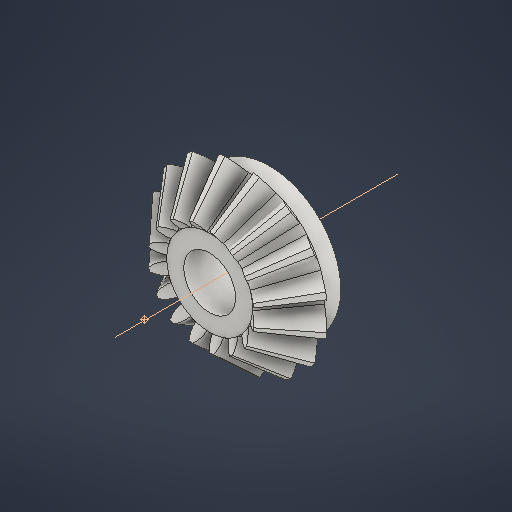
# Autodesk Inventor part: SAFRS-P-0048
Saved by Autodesk Inventor 2026.2 (Build 302298000, 298)
## iProperties
CustomPartVersion: 1
Created: 2025-11-23
Part Number: SAFRS-P-0048
Material: Steel, Mild
Document SubType Name: Modeling
Designer: jaewook
Categories: <?xml version="1.0" encoding="UTF-16"?> <MemberInstance><Categories><FamilyTemplate><FamilyTemplateParameter ValueType="xs:double" Id="1" ObjectReferenceKey="da_z" ObjectType="kUserParameterObject"/><FamilyTemplateParameter ValueType="xs:double" Id="2" ObjectReferenceKey="da_b" ObjectType="kUserParameterObject"/><FamilyTemplateParameter ValueType="xs:double" Id="3" ObjectReferenceKey="da_beta" ObjectType="kUserParameterObject"/><FamilyTemplateParameter ValueType="xs:double" Id="4" ObjectReferenceKey="da_dae" ObjectType="kUserParameterObject"/><FamilyTemplateParameter ValueType="xs:double" Id="5" ObjectReferenceKey="da_ve" ObjectType="kUserParameterObject"/><FamilyTemplateParameter ValueType="xs:double" Id="6" ObjectReferenceKey="da_omega" ObjectType="kUserParameterObject"/><FamilyTemplateParameter ValueType="xs:string" Id="7" ObjectReferenceKey="EAIAABAAAAAAHwAAAAAAAIAAAAAAAAAA" ObjectType="83914240" SubObjectId="SurfaceGeometry"/></FamilyTemplate><ParamToTemplateMap><ParamToTemplate CategoryParameter="//CategoryParameter[@InternalName='046C89C9-8512-4d59-83FE-43B91F4F132A']" TemplateParameter="1"/><ParamToTemplate CategoryParameter="//CategoryParameter[@InternalName='2552DF32-E462-4b46-AEBF-C6C7768E72AC']" TemplateParameter="2"/><ParamToTemplate CategoryParameter="//CategoryParameter[@InternalName='C9EE641D-15FC-4fae-A226-E94C4372FDD7']" TemplateParameter="3"/><ParamToTemplate><ParamToTemplate CategoryParameter="//CategoryParameter[@InternalName='00B6519A-459B-49c7-AD84-2E56D39A5744']" ConstantValue="-0.000000"/></ParamToTemplate><ParamToTemplate><ParamToTemplate CategoryParameter="//CategoryParameter[@InternalName='04B31F0E-C7A6-4894-AA32-9629BEFACF47']" ConstantValue="1.000000"/></ParamToTemplate><ParamToTemplate><ParamToTemplate CategoryParameter="//CategoryParameter[@InternalName='43CBEC2E-7847-49e7-A936-2F7889FCB2D9']" ConstantValue="0.200000"/></ParamToTemplate><ParamToTemplate><ParamToTemplate CategoryParameter="//CategoryParameter[@InternalName='B1EFC894-105D-4ebd-86BF-FA20ED196853']" ConstantValue="0.300000"/></ParamToTemplate><ParamToTemplate><ParamToTemplate CategoryParameter="//CategoryParameter[@InternalName='51175063-3D10-4879-93E8-6246FE8B403D']" ConstantValue="2060000000.000000"/></ParamToTemplate><ParamToTemplate><ParamToTemplate CategoryParameter="//CategoryParameter[@InternalName='A3A52E27-4454-46a9-B0BD-C932399B70AF']" ConstantValue="0.300000"/></ParamToTemplate><ParamToTemplate CategoryParameter="//CategoryParameter[@InternalName='2A200944-5A8C-41ca-B96E-8520D2E510F1']" TemplateParameter="4"/><ParamToTemplate><ParamToTemplate CategoryParameter="//CategoryParameter[@InternalName='1A637F62-92C8-44bc-B81F-10802510B579']" ConstantValue="1.317559"/></ParamToTemplate><ParamToTemplate CategoryParameter="//CategoryParameter[@InternalName='B52DD4BE-6863-48fb-BF58-89EF6F9EC65C']" TemplateParameter="5"/><ParamToTemplate><ParamToTemplate CategoryParameter="//CategoryParameter[@InternalName='3956BFF2-84D2-457d-93C2-9B0613DEBA67']" ConstantValue="0.703377"/></ParamToTemplate><ParamToTemplate CategoryParameter="//CategoryParameter[@InternalName='739CFA02-461B-4bf8-8049-181FCAD8B28F']" TemplateParameter="6"/><ParamToTemplate><ParamToTemplate CategoryParameter="//CategoryParameter[@InternalName='A27E999F-E2CE-4481-8A2A-EBF499C4C3C5']" ConstantValue="-0.000000"/></ParamToTemplate><ParamToTemplate><ParamToTemplate CategoryParameter="//CategoryParameter[@InternalName='9E1B4470-B2D3-4ff1-B813-535BB4CDF51A']" ConstantValue="3520000.000000"/></ParamToTemplate><ParamToTemplate><ParamToTemplate CategoryParameter="//CategoryParameter[@InternalName='F8452263-BFF6-458c-9FB1-07C4B99E95CD']" ConstantValue="11400000.000000"/></ParamToTemplate><ParamToTemplate><ParamToTemplate CategoryParameter="//CategoryParameter[@InternalName='3E3BB259-FD49-497f-8171-6EBC954A3479']" ConstantValue="2.000000"/></ParamToTemplate><ParamToTemplate CategoryParameter="//CategoryParameter[@InternalName='27C3BAF2-7550-4e4b-AE2C-0DB134B7D9B7']" TemplateParameter="7"/></ParamToTemplateMap><Category DisplayName="Gear" InternalName="DC85795E-93AB-48d5-8EEE-5A27447B64BD" Mnemonic="Gear"><CategoryParameter DisplayName="z" InternalName="046C89C9-8512-4d59-83FE-43B91F4F132A" Mnemonic="z"/><CategoryParameter DisplayName="b" InternalName="2552DF32-E462-4b46-AEBF-C6C7768E72AC" Mnemonic="b"/><CategoryParameter DisplayName="||b|" InternalName="C9EE641D-15FC-4fae-A226-E94C4372FDD7" Mnemonic="beta"/><CategoryParameter DisplayName="x" InternalName="00B6519A-459B-49c7-AD84-2E56D39A5744" Mnemonic="x"/><CategoryParameter DisplayName="a*" InternalName="04B31F0E-C7A6-4894-AA32-9629BEFACF47" Mnemonic="a"/><CategoryParameter DisplayName="c*" InternalName="43CBEC2E-7847-49e7-A936-2F7889FCB2D9" Mnemonic="c"/><CategoryParameter DisplayName="r|.f|*" InternalName="B1EFC894-105D-4ebd-86BF-FA20ED196853" Mnemonic="rf"/><CategoryParameter DisplayName="E" InternalName="51175063-3D10-4879-93E8-6246FE8B403D" Mnemonic="E"/><CategoryParameter DisplayName="||m|" InternalName="A3A52E27-4454-46a9-B0BD-C932399B70AF" Mnemonic="mi"/><Category DisplayName="BevelGear" InternalName="0C98F69A-0C2B-4791-B2FE-7691BB227E77" Mnemonic="BevelGear"><CategoryParameter DisplayName="d|.ae|" InternalName="2A200944-5A8C-41ca-B96E-8520D2E510F1" Mnemonic="dae"/><CategoryParameter DisplayName="d|.ai|" InternalName="1A637F62-92C8-44bc-B81F-10802510B579" Mnemonic="dai"/><CategoryParameter DisplayName="A|.e|" InternalName="B52DD4BE-6863-48fb-BF58-89EF6F9EC65C" Mnemonic="ve"/><CategoryParameter DisplayName="A|.i|" InternalName="3956BFF2-84D2-457d-93C2-9B0613DEBA67" Mnemonic="vi"/><CategoryParameter DisplayName="||S|" InternalName="739CFA02-461B-4bf8-8049-181FCAD8B28F" Mnemonic="omega"/><CategoryParameter DisplayName="x|.t|" InternalName="A27E999F-E2CE-4481-8A2A-EBF499C4C3C5" Mnemonic="xt"/><CategoryParameter DisplayName="||s||.Flim|" InternalName="9E1B4470-B2D3-4ff1-B813-535BB4CDF51A" Mnemonic="sFlim"/><CategoryParameter DisplayName="||s||.Hlim|" InternalName="F8452263-BFF6-458c-9FB1-07C4B99E95CD" Mnemonic="sHlim"/><CategoryParameter DisplayName="유형" InternalName="3E3BB259-FD49-497f-8171-6EBC954A3479" Mnemonic="type"/><CategoryParameter DisplayName="PitchDiameter" InternalName="27C3BAF2-7550-4e4b-AE2C-0DB134B7D9B7" Mnemonic="IDS_PITCHDIAM"/></Category></Category></Categories></MemberInstance>
Mass: 60.9118 g
Surface Area: 34.3074 cm^2
Volume: 7.7496 cm^3
Density: 7.86 g/cm^3
Appearance: Steel
Author: jaewook
Title: Bevel Gear 22T
Autodesk Inventor part; units mm, degrees
ref_plane "메쉬 평면2" through (0, 0, 0) normal (0.9807853, 0.1950903, 0) x (0, 0, 1)
sketch "톱니 본체 스케치" plane through (0, 0, 0) normal (1, 0, 0) x (0, 1, 0)
  line L0 (0, 0) -> (8.828697, -13.437043) construction
  line L1 (8.828697, -13.437043) -> (10.976086, -11.719131)
  line L2 (10.976086, -11.719131) -> (0, 0) construction
  line L3 (10, -12.5) -> (0, 0) construction
  line L4 (5.298941, -8.064848) -> (6.587794, -7.033766)
  line L5 (8.828697, -13.437043) -> (5.298941, -8.064848)
  line L6 (10.976086, -11.719131) -> (6.587794, -7.033766)
  line L7 (0, -39.386751) -> (0, 6.564458)
  line L8 (0, -12.5) -> (10.976086, -12.5) construction
  dimension "d0" = 20
  dimension "d1" = 17.65739
  dimension "d2" = 21.95217
  dimension "d3" = 6.4
  dimension "d4" = 11.71913
  constraints: 16 end point, 4 point on line, 3 perpendicular, 2 collinear, 1 horizontal alignment, 1 vertical alignment
  measures "d0" diameter of L3.start L7
  measures "d1" diameter of L0.end L7
  measures "d2" diameter of L1.end L7
  measures "d3" distance between parallel lines of L1 L4
  measures "d4" vertical distance of L1.end L0.start
revolve "톱니 본체" add sketch "톱니 본체 스케치" angle 360 about axis through (0, 0, 0) along (0, 0, 1)
ref_plane "톱니 평면" through (0, 10, -12.5) normal (0, -0.624695, 0.7808688) x (1, 0, 0)
sketch "시작 스케치" plane through (0, 10, -12.5) normal (0, -0.624695, 0.7808688) x (1, 0, 0)
  line L0 (0, -23.505131) -> (0, 10.644758)
  arc A0 (-0.541692, -1.83) -> (-2.580512, 1.849553) centre (-5.33599, -2.081868) ccw
  arc A1 (2.580512, 1.849553) -> (0.541692, -1.83) centre (5.33599, -2.081868) ccw
  line L1 (-0.541692, -1.83) -> (0.541692, -1.83)
  arc A2 (2.580512, 1.849553) -> (-2.580512, 1.849553) centre (0, -12.806248) ccw
  dimension "d7" = 4.80091
  dimension "d8" = 5.33599
  dimension "d9" = 10.72438
  dimension "d57" = 14.88125
  dimension "d58" = 10.97625
  constraints: 6 point on circle, 3 centre point, 3 symmetric about line, 2 end point, 1 coincident, 1 perpendicular, 1 other
  measures "d7" radius of A0
  measures "d8" horizontal distance of point (0, -12.806) A0.centre
  measures "d9" vertical distance of point (0, -12.806) A0.centre
  measures "d57" radius of A2
  measures "d58" distance from line of A2.centre L1
ref_plane "끝 평면" through (0, 5.916056, -7.39507) normal (0, -0.624695, 0.7808688) x (1, 0, 0)
sketch "끝 스케치" plane through (0, 5.916056, -7.39507) normal (0, -0.624695, 0.7808688) x (1, 0, 0)
  line L0 (0, -15.35404) -> (0, 6.953444)
  arc A0 (-0.320468, -1.082638) -> (-1.526645, 1.094206) centre (-3.156802, -1.231645) ccw
  arc A1 (1.526645, 1.094206) -> (0.320468, -1.082638) centre (3.156802, -1.231645) ccw
  line L1 (-0.320468, -1.082638) -> (0.320468, -1.082638)
  arc A2 (1.526645, 1.094206) -> (-1.526645, 1.094206) centre (0, -7.576248) ccw
  dimension "d12" = 2.84024
  dimension "d15" = 3.1568
  dimension "d16" = 6.3446
  dimension "d59" = 8.80383
  dimension "d60" = 6.49361
  constraints: 6 point on circle, 3 centre point, 3 symmetric about line, 2 end point, 1 coincident, 1 other
  measures "d12" radius of A0
  measures "d15" horizontal distance of A0.centre point (0, -7.576)
  measures "d16" vertical distance of A0.centre point (0, -7.576)
  measures "d59" radius of A2
  measures "d60" distance from line of A2.centre L1
loft "Loft" cut profiles "시작 스케치", "끝 스케치"
pattern_circular "Circular Pattern" count 16 over 360 about axis through (0, 0, 0) along (0, 0, 1) of "Loft"
sketch3d "3D 스케치 오른쪽"
ref_plane "끝 평면 오른쪽" through (-1.733589, 5.656358, -7.39507) normal (0.1830551, -0.5972727, 0.7808688) x (0.9561029, 0.2930312, 0)
sketch "끝 스케치 오른쪽" plane through (-1.733589, 5.656358, -7.39507) normal (0.1830551, -0.5972727, 0.7808688) x (0.9561029, 0.2930312, 0)
  arc A0 (-0.320468, -1.082638) -> (-1.526645, 1.094206) centre (-3.156802, -1.231645) ccw
  line L0 (0, -19.389967) -> (0, 10.98936)
  arc A1 (1.526645, 1.094206) -> (0.320468, -1.082638) centre (3.156802, -1.231645) ccw
  line L1 (-0.320468, -1.082638) -> (0.320468, -1.082638)
  arc A2 (1.526645, 1.094206) -> (-1.526645, 1.094206) centre (0, -7.576248) ccw
  dimension "d70" = 3.1568
  dimension "d71" = 6.3446
  dimension "d72" = 2.84024
  dimension "d73" = 6.49361
  dimension "d74" = 8.80383
  constraints: 6 point on circle, 3 centre point, 3 symmetric about line, 2 end point, 1 coincident, 1 perpendicular, 1 other
  measures "d70" horizontal distance of A2.centre A0.centre
  measures "d71" vertical distance of point (0, -7.576) A0.centre
  measures "d72" radius of A0
  measures "d73" distance from line of point (0, -7.576) L1
  measures "d74" radius of A2
feature "로프트 오른쪽" [suppressed]
pattern_circular "원형 패턴 오른쪽" [suppressed]
sketch3d "3D 스케치 왼쪽"
ref_plane "끝 평면 왼쪽" through (1.719596, 5.656358, -7.39034) normal (-0.1816974, -0.5976669, 0.7808843) x (0.9567636, -0.2908668, 0)
sketch "끝 스케치 왼쪽" plane through (1.719596, 5.656358, -7.39034) normal (-0.1816974, -0.5976669, 0.7808843) x (0.9567636, -0.2908668, 0)
  line L0 (0, -33.704724) -> (0, 16.682001)
  arc A0 (-0.320468, -1.082403) -> (-1.526645, 1.094441) centre (-3.156802, -1.23141) ccw
  arc A1 (1.526645, 1.094441) -> (0.320468, -1.082403) centre (3.156802, -1.23141) ccw
  line L1 (-0.320468, -1.082403) -> (0.320468, -1.082403)
  ellipse E0 centre (0, -4.393822) end of major axis (6.587794, -4.393822) minor radius 5.144305
  arc A2 (1.526645, 1.094441) -> (-1.526645, 1.094441) centre (0, -7.576013) ccw
  dimension "d56" = 5.1443
  dimension "d30" = 2.84024
  dimension "d31" = 3.1568
  dimension "d32" = 6.3446
  dimension "d61" = 8.80383
  dimension "d62" = 6.49361
  constraints: 6 point on circle, 3 centre point, 3 symmetric about line, 2 end point, 1 coincident, 2 other
  measures "d30" radius of A0
  measures "d31" horizontal distance of point (0, -7.576) A0.centre
  measures "d32" vertical distance of A0.centre point (0, -7.576)
  measures "d61" radius of A2
  measures "d62" distance from line of point (0, -7.576) L1
feature "로프트 왼쪽" [suppressed]
pattern_circular "원형 패턴 왼쪽" [suppressed]
sketch "본체 스케치" plane through (0, 0, 0) normal (1, 0, 0) x (0, 1, 0)
  line L0 (0, -35.037536) -> (0, -19.530831)
  line L1 (8.828697, -13.437043) -> (5.298941, -8.064848)
  line L2 (5.298941, -8.064848) -> (0, -8.064848)
  line L3 (8.828697, -13.437043) -> (0, -13.437043)
  constraints: 4 end point, 2 perpendicular, 2 point on line
sketch "본체 스케치 outline for 본체 고정" plane through (0, 0, 0) normal (1, 0, 0) x (0, 1, 0)
  line L0 (0, -13.437043) -> (8.828697, -13.437043)
  line L1 (0, -8.064848) -> (0, -13.437043)
  line L2 (5.298941, -8.064848) -> (0, -8.064848)
  line L3 (8.828697, -13.437043) -> (5.298941, -8.064848)
revolve "본체 고정" add sketch "본체 스케치 outline for 본체 고정" angle 360 about axis through (0, 0, 0) along (0, 0, 1)
sketch "Sketch6" plane through (0, 0, 0) normal (1, 0, 0) x (0, 1, 0)
  line L0 (10, -12.5) -> (0, 0)
  line L1 (0, -37.799919) -> (0, 6.299986)
surface revolve "피치 지름" sketch "Sketch6" angle 360 about axis through (0, 0, 0) along (0, 0, 1) shown no curves L0
sketch "스케치8" plane through (0, 0, -8.064848) normal (0, 0, 1) x (1, 0, 0)
  arc A0 (1.708534, 5.015944) -> (0.341039, 5.287955) centre (0, 0) ccw
  circle A1 centre (0, 0) radius 3.2
  dimension "d94" = 6.4
  constraints: 1 centre point, 1 coincident
  measures "d94" diameter of A1
extrude "돌출1" cut sketch "스케치8" against normal blind 10
sketch "스케치9" plane through (0, 0, -13.437043) normal (0, 0, -1) x (-1, 0, 0)
  circle A0 centre (0, 0) radius 3.2
  arc A1 (2.84663, 8.357188) -> (0.568214, 8.810393) centre (0, 0) ccw
  circle A2 centre (0, 0) radius 2
  dimension "d97" = 4
  constraints: 1 centre point, 1 coincident
  measures "d97" diameter of A2
extrude "돌출2" add sketch "스케치9" against normal blind 1
sketch "스케치10" plane through (0, 0, -13.437043) normal (0, 0, -1) x (-1, 0, 0)
  circle A0 centre (0, 0) radius 2
  arc A1 (0.568214, 8.810393) -> (-0.568214, 8.810393) centre (0, 0) ccw
  arc A2 (-0.568214, 8.810393) -> (-2.84663, 8.357188) centre (0, 0) ccw
  arc A3 (-2.84663, 8.357188) -> (-3.896553, 7.922295) centre (0, 0) ccw
  arc A4 (-3.896553, 7.922295) -> (-5.8281, 6.631676) centre (0, 0) ccw
  arc A5 (-5.8281, 6.631676) -> (-6.631676, 5.8281) centre (0, 0) ccw
  arc A6 (-6.631676, 5.8281) -> (-7.922295, 3.896553) centre (0, 0) ccw
  arc A7 (-7.922295, 3.896553) -> (-8.357188, 2.84663) centre (0, 0) ccw
  arc A8 (-8.357188, 2.84663) -> (-8.810393, 0.568214) centre (0, 0) ccw
  arc A9 (-8.810393, 0.568214) -> (-8.810393, -0.568214) centre (0, 0) ccw
  arc A10 (-8.810393, -0.568214) -> (-8.357188, -2.84663) centre (0, 0) ccw
  arc A11 (-8.357188, -2.84663) -> (-7.922295, -3.896553) centre (0, 0) ccw
  arc A12 (-7.922295, -3.896553) -> (-6.631676, -5.8281) centre (0, 0) ccw
  arc A13 (-6.631676, -5.8281) -> (-5.8281, -6.631676) centre (0, 0) ccw
  arc A14 (-5.8281, -6.631676) -> (-3.896553, -7.922295) centre (0, 0) ccw
  arc A15 (-3.896553, -7.922295) -> (-2.84663, -8.357188) centre (0, 0) ccw
  arc A16 (-2.84663, -8.357188) -> (-0.568214, -8.810393) centre (0, 0) ccw
  arc A17 (-0.568214, -8.810393) -> (0.568214, -8.810393) centre (0, 0) ccw
  arc A18 (0.568214, -8.810393) -> (2.84663, -8.357188) centre (0, 0) ccw
  arc A19 (2.84663, -8.357188) -> (3.896553, -7.922295) centre (0, 0) ccw
  arc A20 (3.896553, -7.922295) -> (5.8281, -6.631676) centre (0, 0) ccw
  arc A21 (5.8281, -6.631676) -> (6.631676, -5.8281) centre (0, 0) ccw
  arc A22 (6.631676, -5.8281) -> (7.922295, -3.896553) centre (0, 0) ccw
  arc A23 (7.922295, -3.896553) -> (8.357188, -2.84663) centre (0, 0) ccw
  arc A24 (8.357188, -2.84663) -> (8.810393, -0.568214) centre (0, 0) ccw
  arc A25 (8.810393, -0.568214) -> (8.810393, 0.568214) centre (0, 0) ccw
  arc A26 (8.810393, 0.568214) -> (8.357188, 2.84663) centre (0, 0) ccw
  arc A27 (8.357188, 2.84663) -> (7.922295, 3.896553) centre (0, 0) ccw
  arc A28 (7.922295, 3.896553) -> (6.631676, 5.8281) centre (0, 0) ccw
  arc A29 (6.631676, 5.8281) -> (5.8281, 6.631676) centre (0, 0) ccw
  arc A30 (5.8281, 6.631676) -> (3.896553, 7.922295) centre (0, 0) ccw
  arc A31 (3.896553, 7.922295) -> (2.84663, 8.357188) centre (0, 0) ccw
  arc A32 (2.84663, 8.357188) -> (0.568214, 8.810393) centre (0, 0) ccw
  circle A33 centre (7, 0) radius 1.3
  circle A34 centre (0, 0) radius 3.2
  circle A35 centre (0, 7) radius 1.3
  circle A36 centre (-7, 0) radius 1.3
  circle A37 centre (0, -7) radius 1.3
  dimension "d100" = 2.6
  dimension "d101" = 7
  dimension "d104" = 360
  constraints: 4 centre point, 1 horizontal alignment, 9 other
  measures "d100" diameter of A33
  measures "d101" distance of A34.centre A33.centre
extrude "돌출3" add sketch "스케치10" along normal blind 2 contours A32 A31 A30 A29 A28 A27 A26 A25 A24 A23 A22 A21 A20 A19 A18 A17 A16 A15 A14 A13 A12 A11 A10 A9 A8 A7 A6 A5 A4 A3 A2 A1
sketch "스케치11" plane through (0, 0, -15.437043) normal (0, 0, -1) x (-1, 0, 0)
  circle A0 centre (0, 0) radius 3.2 projected
  circle A1 centre (0, 0) radius 2 projected
extrude "돌출4" add sketch "스케치11" against normal blind 1
sketch "스케치12" plane through (0, 0, -12.437043) normal (0, 0, 1) x (1, 0, 0)
  circle A0 centre (0, 0) radius 3.2 projected
  circle A1 centre (0, 0) radius 2 projected
extrude "돌출5" cut sketch "스케치12" against normal blind 1
equation "\"d0\" = da_de"
equation "\"d1\" = da_dfe"
equation "\"d2\" = da_dae"
equation "\"d3\" = da_b"
equation "\"d4\" = da_ve"
equation "\"d7\" = fd_rr"
equation "\"d8\" = fd_x"
equation "\"d9\" = fd_y"
equation "\"d57\" = 0.5 * fd_dva + 0.3 * da_he"
equation "\"d58\" = 0.5 * fd_dva - 1.12 * da_he"
equation "\"da_teethtype\" = 0"
equation "\"da_b\" = 6.4"
equation "\"da_de\" = 20"
equation "\"da_dae\" = 21.95217"
equation "\"da_dfe\" = 17.65739"
equation "\"da_le\" = 16.00781"
equation "\"da_omega\" = 90deg"
equation "\"da_beta\" = 0"
equation "\"da_delta\" = 38.659808deg"
equation "\"da_alpha\" = 20deg"
equation "\"da_he\" = 2.75"
equation "\"da_ve\" = 11.71913"
equation "\"da_zv\" = 20.489998"
equation "\"fd_loft\" = da_b + 0.05 * da_he"
equation "\"fd_x\" = fd_x1 + fd_x2"
equation "\"fd_y\" = fd_y1 - fd_y2"
equation "\"fd_dd\" = fd_dva - 0.8 * da_he"
equation "\"da_dvw\" = 25.6125"
equation "\"d11\" = fd_loft"
equation "\"da_dm\" = 16.00195"
equation "\"da_x\" = 0"
equation "\"da_m\" = 1.25"
equation "\"d50\" = da_omega"
equation "\"fd_rr\" = 4.800909"
equation "\"fd_dva\" = 28.112497"
equation "\"fd_x1\" = 0.991662"
equation "\"fd_x2\" = 4.344328"
equation "\"fd_y1\" = 12.767796"
equation "\"fd_y2\" = 2.043415"
body "Solid1"
body "Srf1"
